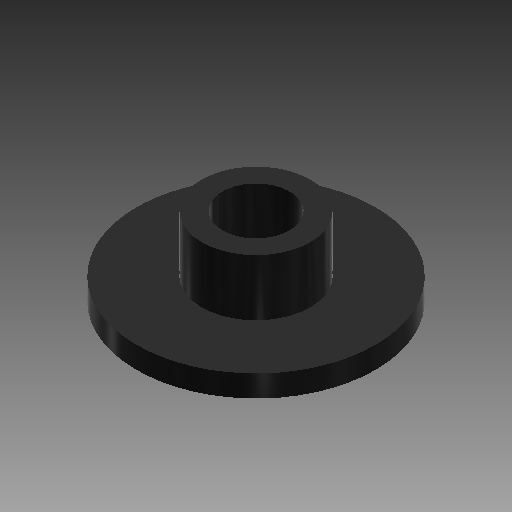
# Autodesk Inventor part: 足首_スペーサ_1_2
Saved by Autodesk Inventor 2018 (Build 220112000, 112)
## iProperties
Category: リンク
Created: 2016-05-01
Part Number: 足首_スペーサ_1_2
Material: アセタール樹脂、黒
Document SubType Name: Modeling
Designer: hiroaki
Density: 1.425 g/cm^3
Appearance: 滑らか - 黒
Mass: 0.16945 g
Surface Area: 2.85429 cm^2
Volume: 0.118912 cm^3
Author: hiroaki
Autodesk Inventor part; units mm, degrees
ref_plane "YZ Plane" through (0, 0, 0) normal (1, 0, 0) x (0, 1, 0)
ref_plane "XZ Plane" through (0, 0, 0) normal (0, 1, 0) x (-1, 0, 0)
ref_plane "XY Plane" through (0, 0, 0) normal (0, 0, 1) x (1, 0, 0)
sketch "スケッチ1" plane through (0, 0, 0) normal (0, 0, 1) x (1, 0, 0)
  line L0 (1.55, 1.8) -> (1.55, -1.8)
  line L1 (1.55, -1.8) -> (5.5, -1.8)
  line L2 (5.5, -1.8) -> (5.5, -0.8)
  line L3 (5.5, -0.8) -> (2.5, -0.8)
  line L4 (2.5, -0.8) -> (2.5, 1.8)
  line L5 (2.5, 1.8) -> (1.55, 1.8)
  line L6 (0, -2.52) -> (0, 2.52) projected
  point P0 (0, 0)
  point P1 (1.55, 0)
  dimension "d0" = 2.5
  dimension "d1" = 1.55
  dimension "d2" = 5.5
  dimension "d3" = 1
  dimension "d7" = 2.6
  constraints: 12 end point, 5 perpendicular, 1 horizontal alignment, 1 midpoint, 1 vertical
  measures "d0" distance from line of point (0, 0) L4
  measures "d1" distance from line of point (0, 0) L0
  measures "d2" distance from line of point (0, 0) L2
  measures "d3" distance of L1.end L2.end
  measures "d7" distance of L3.end L4.end
revolve "回転1" add sketch "スケッチ1" angle 360 about axis through (0, -10, 0) along (0, 1, 0)
